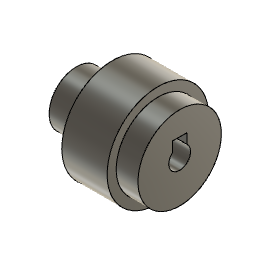
Model 2 (Autodesk Fusion 360 design; units mm, degrees)
Autodesk Fusion 360 part; units mm, degrees
sketch "Sketch1" plane through (0, 0, 0) normal (0, 0, 1) x (1, 0, 0)
  line L0 (0, 0) -> (0, 23)
  line L1 (0, 23) -> (-12, 23)
  line L2 (-12, 23) -> (-12, 28)
  line L3 (-12, 28) -> (-37, 28)
  line L4 (0, 0) -> (-57, 0)
  line L5 (-57, 0) -> (-57, 15)
  line L6 (-57, 15) -> (-37, 15)
  line L7 (-37, 15) -> (-37, 28)
  dimension "d1" = 23
  dimension "d2" = 12
  dimension "d3" = 5
  dimension "d4" = 25
  dimension "d6" = 57
  dimension "d7" = 15
  constraint coincident L0.start L4.start
  constraint vertical L0
  constraint perpendicular L0 L1
  constraint perpendicular L1 L2
  constraint perpendicular L2 L3
  constraint perpendicular L0 L4
  constraint perpendicular L4 L5
  constraint perpendicular L5 L6
  constraint perpendicular L6 L7
  measures "d1" distance of L0.start L0.end
  measures "d2" distance of L0.end L1.end
  measures "d3" distance of L1.end L2.end
  measures "d4" distance of L2.end L3.end
  measures "d6" distance of L0.start L4.end
  measures "d7" distance of L4.end L5.end
revolve "Revolve1" add sketch "Sketch1" angle 360 about axis through (0, 0, 0) along (-1, 0, 0)
sketch "Sketch2" plane through (-57, 0, 0) normal (-1, 0, 0) x (0, -1, 0)
  circle A0 centre (0, 0) radius 15
  line L0 (0, 0) -> (0, -6)
  line L1 (-4, 4.4721) -> (-4, 10)
  line L2 (4, 4.4721) -> (4, 10)
  line L3 (-4, 10) -> (4, 10)
  arc A1 (-4, 4.4721) -> (4, 4.4721) centre (0, 0) ccw
  dimension "d9" = 12
  constraint coincident A0.centre L0.start
  constraint coincident L0.end A1
  constraint vertical L0
  measures "d9" diameter of A1
extrude "Extrude1" cut sketch "Sketch2" against normal through all contours L1 L2 L3 A1
sketch "Sketch3" plane through (-37, 0, 0) normal (-1, 0, 0) x (0, -1, 0)
  circle A0 centre (0, 0) radius 15
  circle A1 centre (0, 0) radius 28
  circle A2 centre (0, 0) radius 21.5 construction
  line L0 (0, 0) -> (0, 21.5) construction
  line L1 (0, 0) -> (21.5, 0) construction
  line L2 (0, 0) -> (0, -21.5) construction
  line L3 (0, 0) -> (-21.5, 0) construction
  circle A3 centre (0, 21.5) radius 2
  circle A4 centre (-21.5, 0) radius 2
  circle A5 centre (0, -21.5) radius 2
  circle A6 centre (21.5, 0) radius 2
  dimension "d18" = 43
  dimension "d19" = 4
  dimension "d21" = 360
  constraint coincident A0.centre A1.centre
  constraint coincident A2 L0.end
  constraint vertical L0
  constraint coincident A2 L1.end
  constraint perpendicular L0 L1
  constraint coincident A2 L2.end
  constraint perpendicular L1 L2
  constraint coincident A2 L3.end
  constraint perpendicular L2 L3
  constraint coincident L0.end A3.centre
  measures "d18" diameter of A2
  measures "d19" diameter of A3
extrude "Extrude2" cut sketch "Sketch3" against normal blind 10 contours A3 | A4 | A5 | A6
